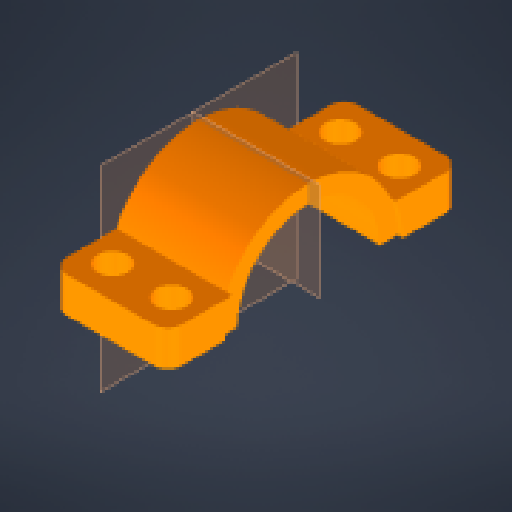
# Autodesk Inventor part: cup
Saved by Autodesk Inventor 2024 (Build 280153000, 153)
## iProperties
Created: 2023-05-16
Part Number: cup
Material: Типовые
Document SubType Name: Modeling
Designer: user
Density: 1 g/cm^3
Appearance: По умолчанию
Author: user
Autodesk Inventor part; units mm, degrees
ref_plane "YZ Plane" through (0, 0, 0) normal (1, 0, 0) x (0, 1, 0)
ref_plane "XZ Plane" through (0, 0, 0) normal (0, 1, 0) x (-1, 0, 0)
ref_plane "XY Plane" through (0, 0, 0) normal (0, 0, 1) x (1, 0, 0)
sketch "Эскиз1" plane through (0, 0, 0) normal (1, 0, 0) x (0, 1, 0)
  line L0 (33, 0) -> (33, -5) projected
  circle A0 centre (12.5, 0) radius 12.5 construction
  arc A1 (1.0436, 5) -> (0, 0) centre (12.5, 0) ccw
  line L1 (0, 0) -> (-8, 0)
  line L2 (-8, 0) -> (-8, 5)
  line L3 (-8, 5) -> (1.0436, 5)
  line L4 (-8, -5) -> (-8, 0) projected
  constraints: 6 end point, 3 point on circle, 2 perpendicular, 1 centre point, 1 collinear, 1 concentric, 1 horizontal
ref_plane "РабПлоскость1" through (16.25, -6, -5) normal (1, 0, 0) x (0, 1, 0)
extrude "Выдавливание1" add sketch "Эскиз1" along normal up to surface (16.25 mm away)
fillet "Сопряжение1" radius 2 2 edges at (0, -8, 2.5) (16.25, -8, 2.5)
sketch "Эскиз2" plane through (16.25, 0, 0) normal (0, 0, -1) x (-1, 0, 0)
  circle A0 centre (12.25, -3.4782) radius 2.15 projected
  circle A1 centre (4, -3.4782) radius 2.15 projected
  point P0 (16.25, 0)
extrude "Выдавливание2" cut sketch "Эскиз2" against normal blind 10
ref_plane "РабПлоскость2" through (0, 12.5, 0) normal (1, 0, 0) x (0, -1, 0)
sketch "Эскиз3" plane through (0, 12.5, 0) normal (1, 0, 0) x (0, -1, 0)
  arc A0 (-12.5, 0) -> (12.5, 0) centre (0, 0) ccw
  circle A1 centre (0, 0) radius 12.5 projected
  circle A2 centre (0, 0) radius 10 projected
  line L0 (-12.5, 0) -> (-10, 0)
  line L1 (12.5, 0) -> (10, 0)
  constraints: 5 point on circle, 4 end point, 1 centre point, 1 coincident, 1 concentric, 1 horizontal, 1 horizontal alignment, 1 point on line
ref_plane "РабПлоскость3" through (15.5, 0, 0) normal (-1, 0, 0) x (0, 0, 1)
extrude "Выдавливание3" add sketch "Эскиз3" along normal up to surface (15.5 mm away) contours L0 A2 L1 A0
ref_plane "РабПлоскость6" through (0, 12.5, 10) normal (0, -1, 0) x (1, 0, 0)
mirror "Зеркальное отражение1" about plane through (0, 12.5, 10) normal (0, -1, 0) of "Выдавливание3", "Выдавливание2", "Сопряжение1", "Выдавливание1"
